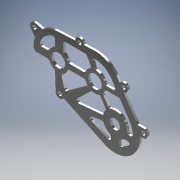
# Autodesk Inventor part: Gearbob Plate
Saved by Autodesk Inventor 2019.4 (Build 234330000, 330)
## iProperties
Created: 2019-11-02
Part Number: Gearbob Plate
Material: Aluminum 6061
Document SubType Name: Modeling
Designer: admin
Density: 2.7 g/cm^3
Appearance: Aluminum - Flat
Mass: 56.197 g
Surface Area: 182.155 cm^2
Volume: 20.8137 cm^3
Author: admin
Autodesk Inventor part; units mm, degrees
ref_plane "YZ Plane" through (0, 0, 0) normal (1, 0, 0) x (0, 1, 0)
ref_plane "XZ Plane" through (0, 0, 0) normal (0, 1, 0) x (-1, 0, 0)
ref_plane "XY Plane" through (0, 0, 0) normal (0, 0, 1) x (1, 0, 0)
sketch "Sketch1" plane through (0, 0, 0) normal (0, 0, 1) x (1, 0, 0)
  circle A0 centre (0, 0) radius 9.5
  circle A1 centre (51.75, 0) radius 9.5
  circle A2 centre (79.8368, -37.996) radius 7
  line L0 (0, 0) -> (51.75, 0) construction
  line L1 (79.8368, -37.996) -> (51.75, 0) construction
  arc A3 (109.0433, -18.7093) -> (64.796, -69.5994) centre (79.8368, -37.996) ccw construction
  arc A4 (49.9384, 37.4562) -> (83.0427, 20.6643) centre (51.75, 0) ccw construction
  arc A5 (-15.0407, -31.6034) -> (-1.6908, 34.9591) centre (0, 0) ccw construction
  line L2 (-1.6908, 34.9591) -> (49.9384, 37.4562)
  line L3 (83.0427, 20.6643) -> (109.0433, -18.7093)
  line L4 (64.796, -69.5994) -> (-15.0407, -31.6034)
  arc A6 (-1.6908, 34.9591) -> (-15.0407, -31.6034) centre (0, 0) ccw
  arc A7 (83.0427, 20.6643) -> (49.9384, 37.4562) centre (51.75, 0) ccw
  arc A8 (64.796, -69.5994) -> (109.0433, -18.7093) centre (79.8368, -37.996) ccw
  dimension "d0" = 19
  dimension "d1" = 19
  dimension "d2" = 14
  dimension "d3" = 51.75
  dimension "d4" = 47.25
  dimension "d5" = 37.996
  dimension "d6" = 70
  dimension "d7" = 75
  dimension "d8" = 70
  constraints: 12 point on circle, 10 end point, 9 centre point, 6 tangent, 4 coincident, 1 horizontal
  measures "d0" diameter of A0
  measures "d1" diameter of A1
  measures "d2" diameter of A2
  measures "d3" distance of L0.start L0.end
  measures "d4" distance of L1.start L0.end
  measures "d5" vertical distance of L1.start L0.end
  measures "d6" diameter of A3
  measures "d7" diameter of A4
  measures "d8" diameter of A5
extrude "Extrusion1" add sketch "Sketch1" along normal blind 3
sketch "Sketch2" plane through (0, 0, 3) normal (0, 0, 1) x (1, 0, 0)
  circle A0 centre (2, -39.7135) radius 2.5
  circle A1 centre (2, -39.7135) radius 6
  circle A2 centre (-33.5852, 23.5166) radius 2.5
  arc A3 (-38.6124, 20.2413) -> (-32.2268, 29.3608) centre (-33.5852, 23.5166) ccw construction
  circle A4 centre (29.75, 36.4798) radius 2.5
  circle A5 centre (29.75, 36.4798) radius 6
  circle A6 centre (91.75, 12.9228) radius 2.5
  circle A7 centre (91.75, 12.9228) radius 6
  circle A8 centre (119.8367, -28.9959) radius 2.5
  arc A9 (119.8367, -22.9959) -> (119.8367, -34.9959) centre (119.8367, -28.9959) ccw construction
  circle A10 centre (79.8368, -37.996) radius 7 projected
  circle A11 centre (51.75, 0) radius 9.5 projected
  circle A12 centre (0, 0) radius 9.5 projected
  line L0 (49.9384, 37.4562) -> (-1.6908, 34.9591) projected
  arc A13 (-1.6908, 34.9591) -> (-15.0407, -31.6034) centre (0, 0) ccw projected
  line L1 (-15.0407, -31.6034) -> (64.796, -69.5994) projected
  arc A14 (64.796, -69.5994) -> (109.0433, -18.7093) centre (79.8368, -37.996) ccw projected
  line L2 (109.0433, -18.7093) -> (83.0427, 20.6643) projected
  arc A15 (83.0427, 20.6643) -> (49.9384, 37.4562) centre (51.75, 0) ccw projected
  arc A16 (-1.6908, 34.9591) -> (-15.0407, -31.6034) centre (0, 0) ccw projected
  line L3 (-32.2268, 29.3608) -> (-22.2268, 27.0364)
  line L4 (-38.6124, 20.2413) -> (-33.008, 11.6394)
  line L5 (-33.5852, 23.5166) -> (0, 0) construction
  line L6 (0, 0) -> (0, 20.8944) construction
  line L7 (119.8367, -22.9959) -> (111.4595, -22.9959)
  line L8 (119.8367, -34.9959) -> (114.7079, -34.9959)
  arc A17 (64.796, -69.5994) -> (109.0433, -18.7093) centre (79.8368, -37.996) ccw projected
  arc A18 (119.8367, -34.9959) -> (119.8367, -22.9959) centre (119.8367, -28.9959) ccw
  arc A19 (-32.2268, 29.3608) -> (-38.6124, 20.2413) centre (-33.5852, 23.5166) ccw
  dimension "d11" = 5
  dimension "d12" = 12
  dimension "d13" = 5
  dimension "d14" = 12
  dimension "d15" = 5
  dimension "d16" = 12
  dimension "d17" = 5
  dimension "d18" = 12
  dimension "d19" = 5
  dimension "d20" = 12
  dimension "d21" = 55
  dimension "d22" = 10
  dimension "d23" = 2
  dimension "d24" = 3
  dimension "d25" = 40
  dimension "d26" = 40
  dimension "d27" = 22
  constraints: 12 centre point, 12 end point, 12 point on circle, 6 tangent, 5 coincident, 2 point on line, 1 equal length, 1 horizontal, 1 parallel, 1 vertical
  measures "d11" diameter of A0
  measures "d12" diameter of A1
  measures "d13" diameter of A2
  measures "d14" diameter of A3
  measures "d15" diameter of A4
  measures "d16" diameter of A5
  measures "d17" diameter of A6
  measures "d18" diameter of A7
  measures "d19" diameter of A8
  measures "d20" diameter of A9
  measures "d21" angle of L6 L5
  measures "d22" horizontal distance of L3.start L3.end
  measures "d23" horizontal distance of point (0, 0) A0.centre
  measures "d24" distance from line of L2 A6.centre
  measures "d25" horizontal distance of A11.centre A6.centre
  measures "d26" horizontal distance of A10.centre A8.centre
  measures "d27" horizontal distance of A11.centre A4.centre
extrude "Extrusion2" add sketch "Sketch2" against normal blind 3 contours A0 L1 A1 | A0 L1 A1 | L4 A19 L3 A13 | A14 L7 A18 L8 | L0 A4 A5 | A5 L0 A4 | L2 A7 | A7 L2
sketch "Sketch3" plane through (0, 0, 3) normal (0, 0, 1) x (1, 0, 0)
  arc A0 (32.2471, 36.6006) -> (27.2529, 36.359) centre (29.75, 36.4798) ccw projected
  arc A1 (-0.2574, -38.6391) -> (4.2574, -40.7878) centre (2, -39.7135) ccw projected
  circle A2 centre (119.8367, -28.9959) radius 2.5 projected
  circle A3 centre (91.75, 12.9228) radius 2.5 projected
  circle A4 centre (-33.5852, 23.5166) radius 2.5 projected
  point P0 (0, 0)
  constraints: 5 coincident
hole "Hole1" at (29.75, 36.4798, 3) at (2, -39.7135, 3) at (119.8367, -28.9959, 3) at (91.75, 12.9228, 3) at (-33.5852, 23.5166, 3) direction (0, 0, -1) diameter 5.5 end through all
sketch "Sketch4" plane through (0, 0, 3) normal (0, 0, 1) x (1, 0, 0)
  arc A0 (-11.1109, -25.1555) -> (0, 27.5) centre (0, 0) ccw construction
  circle A1 centre (51.75, 0) radius 9.5 projected
  arc A2 (51.75, 27.5) -> (74.698, 15.1538) centre (51.75, 0) ccw construction
  circle A3 centre (79.8368, -37.996) radius 7 projected
  arc A4 (100.6986, -24.2198) -> (69.736, -60.8646) centre (79.8368, -37.996) ccw construction
  line L0 (-11.1109, -25.1555) -> (69.736, -60.8646)
  line L1 (100.6986, -24.2198) -> (74.698, 15.1538)
  line L2 (51.75, 27.5) -> (0, 27.5)
  arc A5 (0, 27.5) -> (-11.1109, -25.1555) centre (0, 0) ccw
  arc A6 (74.698, 15.1538) -> (51.75, 27.5) centre (51.75, 0) ccw
  arc A7 (69.736, -60.8646) -> (100.6986, -24.2198) centre (79.8368, -37.996) ccw
  circle A8 centre (0, 0) radius 9.5 projected
  circle A9 centre (0, 0) radius 14.5
  circle A10 centre (51.75, 0) radius 14.5
  circle A11 centre (79.8368, -37.996) radius 17
  line L3 (-13.5981, -5.0342) -> (-27.0353, -5.0342)
  line L4 (-13.5981, 5.0342) -> (-27.0353, 5.0342)
  line L5 (-4.708, 13.7144) -> (-4.708, 27.094)
  line L6 (7.1102, 12.6371) -> (7.1102, 27.5)
  line L7 (47.042, 13.7144) -> (39.6392, 27.5)
  line L8 (51.75, 14.5) -> (46.9446, 27.5)
  line L9 (65.9701, 2.8354) -> (82.8326, 2.8354)
  line L10 (65.9701, -2.8354) -> (86.5773, -2.8354)
  line L11 (58.4979, -12.8342) -> (67.4353, -26.3683)
  line L12 (62.6157, -9.6014) -> (71.9051, -22.9598)
  line L13 (96.4436, -41.631) -> (104.5711, -41.631)
  line L14 (92.1244, -49.7439) -> (101.9045, -49.7439)
  line L15 (74.1845, -54.0288) -> (74.1845, -62.3487)
  line L16 (85.4891, -54.0288) -> (86.42, -62.1136)
  line L17 (63.0853, -35.0998) -> (20.258, -39.0108)
  line L18 (63.3909, -42.301) -> (36.95, -46.3834)
  line L19 (41.5423, -10.2982) -> (8.9587, -34.02)
  line L20 (47.042, -13.7144) -> (20.258, -39.0108)
  line L21 (4.1153, -13.9037) -> (8.9587, -34.02)
  line L22 (-4.708, -13.7144) -> (-4.227, -28.196)
  line L23 (13.9897, 3.8128) -> (37.7603, 3.8128)
  line L24 (37.7603, -3.8128) -> (13.9897, -3.8128)
  dimension "d37" = 55
  dimension "d38" = 55
  dimension "d39" = 50
  dimension "d40" = 5
  dimension "d41" = 5
  dimension "d42" = 10
  constraints: 50 end point, 19 point on circle, 9 point on line, 6 centre point, 6 tangent, 5 parallel, 3 coincident, 3 horizontal, 3 perpendicular, 1 vertical, 32 other
  measures "d37" diameter of A0
  measures "d38" diameter of A2
  measures "d39" diameter of A4
extrude "Extrusion3" cut sketch "Sketch4" against normal blind 3 contours A5 L3 A9 L22 L0 | L21 A9 L24 A10 L19 | A5 L5 A9 L4 | L20 A10 L11 A11 L17 | L18 A11 L15 A7 L0 | L23 A9 L6 L2 L7 A10 | L12 A10 L10 L1 A7 L13 A11 | L16 A11 L14 A7 | L8 L2 A6 L1 L9 A10
fillet "Fillet1" radius 3 31 edges at (8.9587, -34.02, 1.5) (-4.227, -28.196, 1.5) (20.258, -39.0108, 1.5) (4.1153, -13.9037, 1.5) (-4.708, -13.7144, 1.5) (-13.5981, -5.0342, 1.5) (-27.0353, -5.0342, 1.5) (-27.0353, 5.0342, 1.5) (-13.5981, 5.0342, 1.5) (-4.708, 13.7144, 1.5) (-4.708, 27.094, 1.5) (7.1102, 27.5, 1.5) (7.1102, 12.6371, 1.5) (13.9897, 3.8128, 1.5) (37.7603, 3.8128, 1.5) (47.042, 13.7144, 1.5) (39.6392, 27.5, 1.5) (51.75, 14.5, 1.5) (65.9701, 2.8354, 1.5) (82.8326, 2.8354, 1.5) (46.9446, 27.5, 1.5) (104.5711, -41.631, 1.5) (96.4436, -41.631, 1.5) (71.9051, -22.9598, 1.5) (62.6157, -9.6014, 1.5) (65.9701, -2.8354, 1.5) (86.5773, -2.8354, 1.5) (74.1845, -62.3487, 1.5) (36.95, -46.3834, 1.5) (63.3909, -42.301, 1.5) (74.1845, -54.0288, 1.5)
fillet "Fillet2" radius 2 4 edges at (86.42, -62.1136, 1.5) (85.4891, -54.0288, 1.5) (92.1244, -49.7439, 1.5) (101.9045, -49.7439, 1.5)
sketch "Sketch5" plane through (0, 0, 3) normal (0, 0, 1) x (1, 0, 0)
  line L0 (-4.6439, -15.6435) -> (-4.3856, -23.4225) projected
  line L1 (-4.3856, -23.4225) -> (-3.9384, -36.8873)
  line L2 (-3.4177, -37.1351) -> (-15.0407, -31.6034) projected
  line L3 (-4.3856, -23.4225) -> (9.0867, -23.4225) construction
  line L4 (-23.1452, -5.0342) -> (-15.5468, -5.0342) projected
  line L5 (-4.3856, -23.4225) -> (-23.1452, -5.0342)
  line L6 (-23.1452, -5.0342) -> (-43.6946, -5.0342)
  line L7 (-43.6946, -5.0342) -> (-26.4019, -52.6699)
  line L8 (-3.9384, -36.8873) -> (-26.4019, -52.6699)
  point P0 (0, 0)
  constraints: 12 end point, 2 horizontal, 1 collinear, 1 equal length, 1 point on line
extrude "Extrusion4" cut sketch "Sketch5" against normal blind 10
fillet "Fillet3" radius 5 2 edges at (-3.9384, -36.8873, 1.5) (-34.6361, -5.0342, 1.5)
body "Solid1"
